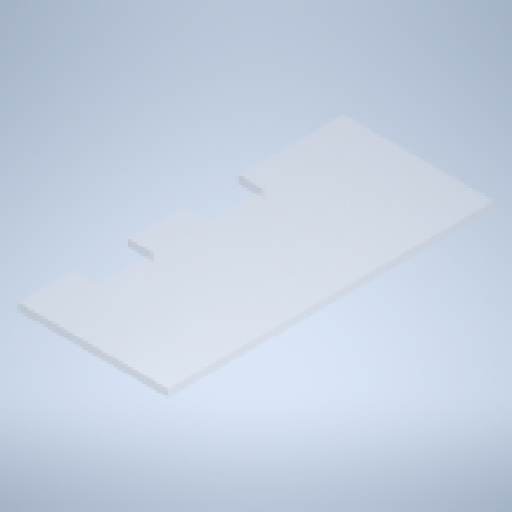
# Autodesk Inventor part: 라즈베리파이_SMPS 격리판
Saved by Autodesk Inventor 2024 (Build 280153000, 153)
## iProperties
Created: 2024-04-10
Part Number: 라즈베리파이_SMPS 격리판
Material: PMMA 플라스틱
Document SubType Name: Modeling
Designer: kkamin5
Mass: 39.204 g
Surface Area: 149 cm^2
Volume: 33 cm^3
Density: 1.188 g/cm^3
Appearance: 폴리카보네이트 - 선명
Author: kkamin5
Autodesk Inventor part; units mm, degrees
ref_plane "YZ Plane" through (0, 0, 0) normal (1, 0, 0) x (0, 1, 0)
ref_plane "XZ Plane" through (0, 0, 0) normal (0, 1, 0) x (-1, 0, 0)
ref_plane "XY Plane" through (0, 0, 0) normal (0, 0, 1) x (1, 0, 0)
sketch "스케치1" plane through (0, 0, 0) normal (0, 1, 0) x (-1, 0, 0)
  line L0 (30, 50) -> (-30, 50)
  line L1 (-30, 50) -> (-30, -80)
  line L2 (-30, -80) -> (30, -80)
  line L3 (30, -80) -> (30, 50)
  point P0 (0, 0)
  dimension "d0" = 130
  dimension "d1" = 60
  dimension "d2" = 30
  dimension "d3" = 50
  constraints: 8 end point, 2 parallel, 1 horizontal, 1 perpendicular
  measures "d0" distance of L0.end L1.end
  measures "d1" distance of L1.end L2.end
  measures "d2" distance from line of point (0, 0) L3
  measures "d3" distance from line of point (0, 0) L0
extrude "돌출1" add sketch "스케치1" along normal blind 3
sketch "스케치2" plane through (0, 3, 0) normal (0, 1, 0) x (1, 0, 0)
  line L0 (-30, 80) -> (-30, -50) projected
  line L1 (-10, 54) -> (-30, 54)
  line L2 (-30, 54) -> (-30, 28)
  line L3 (-30, 28) -> (-10, 28)
  line L4 (-10, 28) -> (-10, 54)
  line L5 (-10, 2) -> (-30, 2)
  line L6 (-30, 2) -> (-30, -24)
  line L7 (-30, -24) -> (-10, -24)
  line L8 (-10, -24) -> (-10, 2)
  line L9 (-30, -50) -> (30, -50) projected
  point P0 (0, 0)
  dimension "d6" = 26
  dimension "d7" = 26
  dimension "d8" = 26
  dimension "d9" = 26
  dimension "d10" = 20
  constraints: 16 end point, 4 parallel, 3 point on line, 2 horizontal, 2 perpendicular
  measures "d6" distance between parallel lines of L7 L9
  measures "d7" distance between parallel lines of L7 L5
  measures "d8" distance between parallel lines of L5 L3
  measures "d9" distance between parallel lines of L3 L1
  measures "d10" distance between parallel lines of L0 L8
extrude "돌출2" cut sketch "스케치2" against normal blind 10
equation "\"d7\" = d6"
equation "\"d8\" = d7"
equation "\"d9\" = d8"
